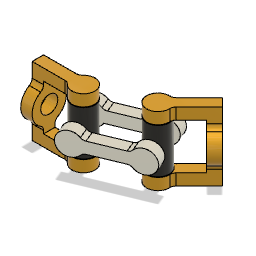
cardan_joint (Autodesk Fusion 360 design; units mm, degrees)
Autodesk Fusion 360 part; units mm, degrees
sketch "Sketch1" plane through (0, 0, 0) normal (0, 0, 1) x (1, 0, 0) in component "Yoke"
  line L0 (5, 30) -> (-35, 30)
  line L1 (-35, 30) -> (-35, -30)
  line L2 (-35, -30) -> (5, -30)
  line L3 (5, 20) -> (-25, 20)
  line L4 (-25, 20) -> (-25, -20)
  line L5 (-25, -20) -> (5, -20)
  line L6 (5, 20) -> (5, 30)
  line L7 (5, -20) -> (5, -30)
  dimension "d1" = 40
  dimension "d2" = 60
  dimension "d5" = -10
  dimension "d8" = 40
  dimension "d9" = 25
  dimension "d10" = 20
  dimension "d212" = 40
  dimension "d213" = 30
  constraint perpendicular L0 L1
  constraint parallel L0 L2
  constraint horizontal L0
  constraint perpendicular L0 L6
  constraint perpendicular L2 L7
  measures "d1" distance of L1.end L2.end
  measures "d2" distance of L0.end L1.end
  measures "d8" distance of L0.start L0.end
  measures "d9" distance of origin L4
  measures "d10" distance of origin L5
  measures "d212" distance of L3.end L4.end
  measures "d213" distance of origin L2
extrude "Extrude1" add sketch "Sketch1" along normal mid plane 10 makes body 1 in component "Yoke"
sketch "Sketch2" plane through (-35, 0, 0) normal (-1, 0, 0) x (0, 0, 1) in component "Yoke"
  line L0 (-5, -30) -> (5, -30)
  line L1 (5, -30) -> (5, 30)
  line L2 (5, 30) -> (-5, 30)
  line L3 (-5, 30) -> (-5, -30)
  circle A0 centre (0, 0) radius 15
  circle A1 centre (0, 0) radius 7.5
  dimension "d11" = 30
  dimension "d12" = 15
  constraint coincident A0.centre A1.centre
  measures "d11" diameter of A0
  measures "d12" diameter of A1
extrude "Extrude2" add sketch "Sketch2" against normal blind 10 contours L3 A0 A1 | L1 L3 A0 A1 | L1 A0 A1 | L1 L3 A0 A1 bodies 1 in component "Yoke"
extrude "Extrude3" cut sketch "Sketch2" against normal blind 44 contours L3 A1 | L1 L3 A1 | L1 A1 bodies 1 in component "Yoke"
fillet "Fillet1" radius 5 4 edges at (-30, 14.1421, 5) (-30, 14.1421, -5) (-30, -14.1421, -5) (-30, -14.1421, 5) on bodies 1 in component "Yoke"
cylinder "CylinderPrimitive1" add diameter 20 height -10 placed x (1, 0, 0) y (0, 0, -1) z (0, 1, 0) at (5, 30, 0) bodies 1 in component "Yoke"
mirror "Mirror1" about plane through (0, 0, 0) normal (0, 1, 0) of "CylinderPrimitive1" in component "Yoke"
cylinder "CylinderPrimitive2" add diameter 10 height 5 placed x (1, 0, 0) y (0, 0, -1) z (0, 1, 0) at (5, -20, 0) bodies 1 in component "Yoke"
mirror "Mirror2" about plane through (0, 0, 0) normal (0, 1, 0) of "CylinderPrimitive2" in component "Yoke"
fillet "Fillet2" radius 5 4 edges at (-3.6603, 25, 5) (-3.6603, 25, -5) (-3.6603, -25, -5) (-3.6603, -25, 5) on bodies 1 in component "Yoke"
fillet "Fillet4" radius 0.5 4 edges at (0.3384, 15, 1.8081) (0.3384, -15, 1.8081) (0.3384, -20, -1.8081) (0.3384, 20, 1.8081) on bodies 1 in component "Yoke"
cylinder "CylinderPrimitive1'" add diameter 20 height 40 placed x (1, 0, 0) y (0, 0, -1) z (0, 1, 0) at (5, -20, 0) separate body makes body 2 in component "Pin"
sketch "Sketch4" plane through (0, 0, 0) normal (0, 0, 1) x (1, 0, 0) in component "Pin"
  line L0 (-5, -20) -> (15, -20)
  line L1 (15, 20) -> (-5, 20)
  line L2 (15, -20) -> (15, 20)
  line L3 (-5, -20) -> (-5, 20)
  circle A0 centre (5, 0) radius 5
  dimension "d32" = 10
  measures "d32" diameter of A0
extrude "Extrude3'" cut sketch "Sketch4" along normal mid plane 54 contours A0 bodies 2 in component "Pin"
combine "Combine3" operation cut target body 2 tool bodies 1 keep tools in component "Pin"
fillet "Fillet3" [suppressed] in component "Yoke"
fillet "Fillet2'" radius 0.5 4 edges at (-4.3233, 20, 3.6162) (0, 0, 8.6603) (0, 0, -8.6603) (-4.3233, -20, -3.6162) on bodies 2 in component "Pin"
sketch "Sketch1 (2)" plane through (0, 0, 0) normal (0, 0, 1) x (1, 0, 0) in component "Center Block"
  spline S0 degree 3 poles (10, 0) (10, -0.271) (9.9778, -0.5419) (9.8647, -1.233) (9.7406, -1.6443) (9.372, -2.4747) (9.1118, -2.8851) (8.41, -3.7056) (7.9384, -4.0912) (6.6845, -4.7785) (5.8452, -5.0001) (4.2461, -4.9999) (3.4969, -4.8248) (2.0792, -4.144) (1.4353, -3.6013) (0.4145, -2.1937) (0.0731, -1.2824) (-0.0446, 0.5205) (0.1243, 1.379) (0.7453, 2.7036) (1.1235, 3.2208) (2.0369, 4.0745) (2.5704, 4.4158) (3.6824, 4.8558) (4.2487, 4.9763) (5.7266, 5.0292) (6.636, 4.8057) (8.0664, 4.0205) (8.6298, 3.5178) (9.6523, 2.0929) (10, 1.0594) (10, 0) knots 0 0 0 0 0.077638 0.077638 0.201859 0.201859 0.346163 0.346163 0.526489 0.526489 0.768843 0.768843 0.98465 0.98465 1.23151 1.23151 1.506411 1.506411 1.749621 1.749621 1.939638 1.939638 2.125125 2.125125 2.289237 2.289237 2.548932 2.548932 2.771597 2.771597 3.075124 3.075124 3.075124 3.075124
  line L0 (10, 0) -> (10, -0.271)
  line L1 (10, -0.271) -> (9.9778, -0.5419)
  line L2 (9.9778, -0.5419) -> (9.8647, -1.233)
  line L3 (9.8647, -1.233) -> (9.7406, -1.6443)
  line L4 (9.7406, -1.6443) -> (9.372, -2.4747)
  line L5 (9.372, -2.4747) -> (9.1118, -2.8851)
  line L6 (9.1118, -2.8851) -> (8.41, -3.7056)
  line L7 (8.41, -3.7056) -> (7.9384, -4.0912)
  line L8 (7.9384, -4.0912) -> (6.6845, -4.7785)
  line L9 (6.6845, -4.7785) -> (5.8452, -5.0001)
  line L10 (5.8452, -5.0001) -> (4.2461, -4.9999)
  line L11 (4.2461, -4.9999) -> (3.4969, -4.8248)
  line L12 (3.4969, -4.8248) -> (2.0792, -4.144)
  line L13 (2.0792, -4.144) -> (1.4353, -3.6013)
  line L14 (1.4353, -3.6013) -> (0.4145, -2.1937)
  line L15 (0.4145, -2.1937) -> (0.0731, -1.2824)
  line L16 (0.0731, -1.2824) -> (-0.0446, 0.5205)
  line L17 (-0.0446, 0.5205) -> (0.1243, 1.379)
  line L18 (0.1243, 1.379) -> (0.7453, 2.7036)
  line L19 (0.7453, 2.7036) -> (1.1235, 3.2208)
  line L20 (1.1235, 3.2208) -> (2.0369, 4.0745)
  line L21 (2.0369, 4.0745) -> (2.5704, 4.4158)
  line L22 (2.5704, 4.4158) -> (3.6824, 4.8558)
  line L23 (3.6824, 4.8558) -> (4.2487, 4.9763)
  line L24 (4.2487, 4.9763) -> (5.7266, 5.0292)
  line L25 (5.7266, 5.0292) -> (6.636, 4.8057)
  line L26 (6.636, 4.8057) -> (8.0664, 4.0205)
  line L27 (8.0664, 4.0205) -> (8.6298, 3.5178)
  line L28 (8.6298, 3.5178) -> (9.6523, 2.0929)
  line L29 (9.6523, 2.0929) -> (10, 1.0594)
  line L30 (10, 1.0594) -> (10, 0)
  circle A0 centre (5, 0) radius 5 construction
  circle A1 centre (5, 0) radius 10
  dimension "d43" = 20
  dimension "d83" = 0
  dimension "d84" = 0
  dimension "d85" = 0
  dimension "d86" = 0
  constraint coincident S0.start S0.end
  constraint coincident S0.start A0
  constraint coincident origin A0
  constraint concentric A0 A1
  measures "d43" diameter of A1
extrude "Extrude1'" add sketch "Sketch1 (2)" along normal mid plane 25 separate body contours S0 L0 L1 L2 | S0 makes body 3 in component "Center Block"
extrude "Extrude2'" add sketch "Sketch1 (2)" along normal blind 10 from surface at 12.5 contours S0 L0 L1 L2 | S0 | S0 L28 L29 L30 | S0 L2 L3 L4 | S0 L26 L27 L28 | S0 L4 L5 L6 | S0 L24 L25 L26 | S0 L6 L7 L8 | S0 L22 L23 L24 | S0 L8 L9 L10 | S0 L20 L21 L22 | S0 L10 L11 L12 | S0 L18 L19 L20 | S0 L12 L13 L14 | S0 L16 L17 L18 | S0 L14 L15 L16 | A1 bodies 3 in component "Center Block"
mirror "Mirror1'" about plane through (0, 0, 0) normal (0, 0, 1) of "Extrude2'" in component "Center Block"
copy_body "CopyPasteBodies1" bodies 3 makes body 4 in component "Center Block"
move_body "Move1" bodies 4 to x (1, 0, 0) y (0, 1, 0) z (0, 0, 1) at (50, 0, 0) in component "Center Block"
sketch "Sketch2 (2)" plane through (0, 0, 22.5) normal (0, 0, 1) x (1, 0, 0) in component "Center Block"
  circle A0 centre (5, 0) radius 10
  line L0 (5, 5) -> (55, 5)
  line L1 (55, 5) -> (55, -5)
  line L2 (55, -5) -> (5, -5)
  line L3 (5, -5) -> (5, 5)
  dimension "d50" = 10
  dimension "d51" = 50
  dimension "d52" = 5
  constraint horizontal L0
  constraint vertical L1
  constraint horizontal L2
  constraint vertical L3
  constraint coincident A0.centre L3
  measures "d50" distance of L0.start L2.end
  measures "d51" distance of L0.start L0.end
  measures "d52" distance of A0.centre L0
extrude "Extrude3''" add sketch "Sketch2 (2)" against normal blind 10 contours A0 L0 L2 L3 | A0 L0 L1 L2 picked at (8.3333, 0) bodies 3 in component "Center Block"
mirror "Mirror2'" about plane through (0, 0, 0) normal (0, 0, 1) of "Extrude3''" in component "Center Block"
combine "Combine1" operation add target body 4 tool bodies 3 in component "Center Block"
fillet "Fillet1'" radius 5 6 edges at (13.6603, 5, 17.5) (46.3397, 5, 17.5) (46.3397, 5, -17.5) (13.6603, 5, -17.5) (13.6603, -5, 17.5) (46.3397, -5, 17.5) on bodies 4 in component "Center Block"
cylinder "CylinderPrimitive1''" add diameter 15 height 40 placed x (0, 0, 1) y (0, 1, 0) z (-1, 0, 0) at (-35, 0, 0) separate body makes body 5 in component "Component"
component "Yoke" placed x (1, 0, 0) y (0, 1, 0) z (0, 0, 1) at (-10, 0, 0)
component "Yoke" placed x (-0.707107, 0, 0.707107) y (0, 1, 0) z (-0.707107, 0, -0.707107) at (44.7311, 0, -22.6658)
component "Pin" placed x (0.92388, 0, -0.382683) y (0, 1, 0) z (0.382683, 0, 0.92388) at (-9.6194, 0, 1.9134)
component "Pin" placed x (0.92388, 0, -0.382683) y (0, -1, 0) z (-0.382683, 0, -0.92388) at (36.5762, 0, -17.2168)
component "Center Block" placed x (0.92388, 0, -0.382683) y (0, 1, 0) z (0.382683, 0, 0.92388) at (-9.4368, 0, 2.3541)
component "Component" placed x (1, 0, 0) y (0, 1, 0) z (0, 0, 1) at (0, 0, 0)
component "Component" placed x (0.707107, 0, -0.707107) y (0, 1, 0) z (0.707107, 0, 0.707107) at (115.4418, 0, -93.3765)
